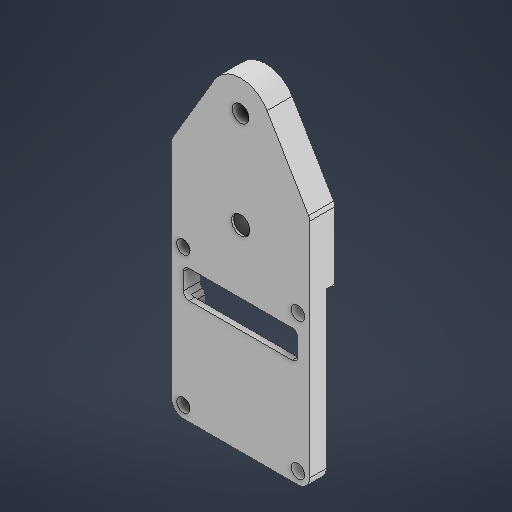
# Autodesk Inventor part: servo_side_plate2
Saved by Autodesk Inventor 2026 (Build 300175000, 175)
## iProperties
Created: 2025-12-05
Part Number: servo_side_plate2
Material: Generic
Document SubType Name: Modeling
Designer: numai
Density: 1 g/cm^3
Appearance: Default
Author: numai
Autodesk Inventor part; units mm, degrees
ref_plane "YZ Plane" through (0, 0, 0) normal (1, 0, 0) x (0, 1, 0)
ref_plane "XZ Plane" through (0, 0, 0) normal (0, 1, 0) x (-1, 0, 0)
ref_plane "XY Plane" through (0, 0, 0) normal (0, 0, 1) x (1, 0, 0)
sketch "スケッチ1" plane through (0, 0, 0) normal (0, 0, 1) x (1, 0, 0)
  circle A0 centre (0, 12.5) radius 5 construction
  line L0 (12.16, 19.2887) -> (12.16, 6.89) construction
  arc A1 (12.16, 19.2887) -> (11.7792, 20.2079) centre (10.86, 19.2887) ccw construction
  line L1 (9.9579, 22.0292) -> (11.7792, 20.2079) construction
  arc A2 (9.9579, 22.0292) -> (9.0387, 22.41) centre (9.0387, 21.11) ccw construction
  line L2 (0.95, 22.41) -> (9.0387, 22.41) construction
  line L3 (0.95, 19.61) -> (0.95, 22.41) construction
  arc A3 (-0.95, 19.61) -> (0.95, 19.61) centre (0, 19.61) ccw construction
  line L4 (-0.95, 22.41) -> (-0.95, 19.61) construction
  line L5 (-9.0387, 22.41) -> (-0.95, 22.41) construction
  arc A4 (-9.0387, 22.41) -> (-9.9579, 22.0292) centre (-9.0387, 21.11) ccw construction
  line L6 (-11.7792, 20.2079) -> (-9.9579, 22.0292) construction
  arc A5 (-11.7792, 20.2079) -> (-12.16, 19.2887) centre (-10.86, 19.2887) ccw construction
  line L7 (-12.16, 6.89) -> (-12.16, 19.2887) construction
  line L8 (-12.16, 6.89) -> (-9.9756, 6.89) construction
  arc A6 (-9.8028, 6.7907) -> (-9.9756, 6.89) centre (-9.9756, 6.69) ccw construction
  arc A7 (-9.8028, 6.7907) -> (-6.5643, 3.2479) centre (0, 12.5) ccw construction
  arc A8 (-6.48, 3.0847) -> (-6.5643, 3.2479) centre (-6.68, 3.0847) ccw construction
  line L9 (-6.48, 3.0847) -> (-6.48, 1.39) construction
  arc A9 (-6.68, 1.19) -> (-6.48, 1.39) centre (-6.68, 1.39) ccw construction
  line L10 (-6.68, 1.19) -> (6.68, 1.19) projected
  arc A10 (6.48, 1.39) -> (6.68, 1.19) centre (6.68, 1.39) ccw construction
  line L11 (6.48, 1.39) -> (6.48, 3.0847) construction
  arc A11 (6.5643, 3.2479) -> (6.48, 3.0847) centre (6.68, 3.0847) ccw construction
  arc A12 (6.5643, 3.2479) -> (9.8028, 6.7907) centre (0, 12.5) ccw construction
  arc A13 (9.9756, 6.89) -> (9.8028, 6.7907) centre (9.9756, 6.69) ccw construction
  line L12 (9.9756, 6.89) -> (12.16, 6.89) construction
  arc A14 (12.36, 19.2887) -> (12.1513, 20.052) centre (10.86, 19.2887) ccw projected
  arc A15 (-12.1513, 20.052) -> (-12.36, 19.2887) centre (-10.86, 19.2887) ccw projected
  line L13 (12.36, 19.2887) -> (12.36, -20.5) projected
  line L14 (-12.36, -20.5) -> (-12.36, 19.2887) projected
  line L15 (-12.36, 6.89) -> (-9.86, 6.89)
  line L16 (12.36, 6.89) -> (9.86, 6.89)
  arc A16 (-9.86, 6.89) -> (9.86, 6.89) centre (0, 12.5) ccw
  circle A17 centre (0, 12.5) radius 5.2
  arc A18 (4.7347, 32.5987) -> (-4.7347, 32.5987) centre (0, 29.8) ccw projected
  line L17 (-12.1513, 20.052) -> (-4.7347, 32.5987) projected
  circle A19 centre (0, 29.8) radius 1.5
  line L18 (4.7347, 32.5987) -> (12.1513, 20.052) projected
  circle A20 centre (0, 29.8) radius 1.5 construction
  point P0 (0, 0)
  point P1 (-11.1384, 22.2293)
  point P2 (11.1384, 22.2293)
  point P3 (-0.8807, 1.19)
  point P4 (0.8807, 1.19)
  dimension "d0" = 10.4
  constraints: 4 end point, 4 point on line, 3 centre point, 3 point on circle, 2 coincident, 2 concentric, 2 horizontal
  measures "d0" diameter of A17
extrude "押し出し1" add sketch "スケッチ1" along normal blind 1.5 contours A16 L15 L14 A15 L17 A18 L18 A14 L13 L16 L10
sketch "スケッチ2" plane through (0, 0, 1.5) normal (0, 0, 1) x (1, 0, 0)
  arc A0 (-9.86, 6.89) -> (-0.8807, 1.19) centre (0, 12.5) ccw projected
  line L0 (9.1914, -4.7213) -> (9.25, -4.7213) projected
  ellipse E0 centre (9.05, -4.9213) end of major axis (9.05, -4.6384) minor radius 0.2 (9.25, -4.9213) -> (9.1914, -4.7213) ccw projected
  line L1 (9.25, -4.9213) -> (9.25, -17.11) projected
  arc A1 (9.05, -17.31) -> (9.25, -17.11) centre (9.05, -17.11) ccw projected
  line L2 (9.05, -17.31) -> (-9.05, -17.31) projected
  arc A2 (-9.25, -17.11) -> (-9.05, -17.31) centre (-9.05, -17.11) ccw projected
  line L3 (-9.25, -17.11) -> (-9.25, -4.9213) projected
  ellipse E1 centre (-9.05, -4.9213) end of major axis (-9.05, -5.2041) minor radius 0.2 (-9.1914, -4.7213) -> (-9.25, -4.9213) ccw projected
  line L4 (-9.25, -4.7213) -> (-9.1914, -4.7213) projected
  ellipse E2 centre (-9.25, -3.0242) end of major axis (-9.25, -4.7213) minor radius 1.2 (-10.45, -3.0242) -> (-9.25, -4.7213) ccw projected
  line L5 (-10.45, 0.19) -> (-10.45, -3.0242) projected
  arc A3 (-9.25, 1.39) -> (-10.45, 0.19) centre (-9.25, 0.19) ccw projected
  line L6 (-6.68, 1.39) -> (-9.25, 1.39) projected
  line L7 (-6.68, 3.0847) -> (-6.68, 1.39) projected
  arc A4 (-9.9756, 6.69) -> (-6.68, 3.0847) centre (0, 12.5) ccw construction
  line L8 (-12.16, 6.69) -> (-9.9756, 6.69) construction
  line L9 (-12.16, -20.5) -> (-12.16, 6.69) construction
  arc A5 (-12.16, -20.5) -> (-10.25, -22.41) centre (-10.25, -20.5) ccw construction
  line L10 (10.25, -22.41) -> (-10.25, -22.41) construction
  arc A6 (10.25, -22.41) -> (12.16, -20.5) centre (10.25, -20.5) ccw construction
  line L11 (12.16, 6.69) -> (12.16, -20.5) construction
  line L12 (9.9756, 6.69) -> (12.16, 6.69) construction
  arc A7 (6.68, 3.0847) -> (9.9756, 6.69) centre (0, 12.5) ccw construction
  line L13 (6.68, 1.39) -> (6.68, 3.0847) projected
  line L14 (9.25, 1.39) -> (6.68, 1.39) projected
  arc A8 (10.45, 0.19) -> (9.25, 1.39) centre (9.25, 0.19) ccw projected
  line L15 (10.45, -3.0242) -> (10.45, 0.19) projected
  ellipse E3 centre (9.25, -3.0242) end of major axis (9.25, -4.7213) minor radius 1.2 (9.25, -4.7213) -> (10.45, -3.0242) ccw projected
  circle A9 centre (10.25, 4) radius 0.7835 construction
  circle A10 centre (10.25, -20.5) radius 0.7835 construction
  circle A11 centre (-10.25, -20.5) radius 0.7835 construction
  circle A12 centre (-10.25, 4) radius 0.7835 construction
  arc A13 (-12.36, -20.5) -> (-10.25, -22.61) centre (-10.25, -20.5) ccw projected
  line L16 (-12.36, 6.69) -> (-12.36, -20.5) projected
  line L17 (-10.25, -22.61) -> (10.25, -22.61) projected
  arc A14 (10.25, -22.61) -> (12.36, -20.5) centre (10.25, -20.5) ccw projected
  line L18 (12.36, -20.5) -> (12.36, 6.69) projected
  line L19 (12.36, 6.69) -> (12.36, 19.2887) projected
  line L20 (-12.36, 19.2887) -> (-12.36, 6.69) projected
  circle A15 centre (-10.25, 4) radius 1.2
  circle A16 centre (-10.25, -20.5) radius 1.2
  circle A17 centre (10.25, -20.5) radius 1.2
  circle A18 centre (10.25, 4) radius 1.2
  line L21 (-6.68, 3.0847) -> (-6.68, 3.3311)
  line L22 (6.68, 3.0847) -> (6.68, 3.3311)
  line L23 (-6.68, 1.39) -> (6.68, 1.39)
  line L24 (9.86, 6.89) -> (12.36, 6.89) projected
  line L25 (12.36, 6.89) -> (12.36, 19.2887) projected
  arc A19 (12.36, 19.2887) -> (12.1513, 20.052) centre (10.86, 19.2887) ccw projected
  line L26 (12.1513, 20.052) -> (4.7347, 32.5987) projected
  arc A20 (4.7347, 32.5987) -> (-4.7347, 32.5987) centre (0, 29.8) ccw projected
  line L27 (-4.7347, 32.5987) -> (-12.1513, 20.052) projected
  arc A21 (-12.1513, 20.052) -> (-12.36, 19.2887) centre (-10.86, 19.2887) ccw projected
  line L28 (-12.36, 19.2887) -> (-12.36, 6.89) projected
  line L29 (-12.36, 6.89) -> (-9.86, 6.89) projected
  line L30 (-0.8807, 1.19) -> (0.8807, 1.19) projected
  arc A22 (0.8807, 1.19) -> (9.86, 6.89) centre (0, 12.5) ccw projected
  circle A23 centre (0, 12.5) radius 5.2 projected
  circle A24 centre (0, 29.8) radius 1.5 projected
  arc A25 (-10.25, -2.81) -> (-9.25, -3.81) centre (-9.25, -2.81) ccw projected
  line L31 (-10.25, -3.0242) -> (-10.25, 0.19) projected
  arc A26 (-9.25, 1.19) -> (-10.25, 0.19) centre (-9.25, 0.19) ccw projected
  line L32 (-9.25, 1.19) -> (-6.68, 1.19) projected
  line L33 (-6.68, 1.19) -> (6.68, 1.19) projected
  line L34 (6.68, 1.19) -> (9.25, 1.19) projected
  arc A27 (10.25, 0.19) -> (9.25, 1.19) centre (9.25, 0.19) ccw projected
  line L35 (10.25, 0.19) -> (10.25, -3.0242) projected
  arc A28 (9.25, -3.81) -> (10.25, -2.81) centre (9.25, -2.81) ccw projected
  line L36 (-9.25, -3.81) -> (9.25, -3.81) projected
  line L37 (-9.25, -4.9213) -> (-9.25, -3.81)
  line L38 (9.25, -4.9213) -> (9.25, -3.81)
  point P0 (0, 0)
  point P1 (12.36, 6.89)
  point P2 (-2.2934, 1.39)
  point P3 (2.2934, 1.39)
  point P4 (2.2934, 1.39)
  dimension "d3" = 2.4
  constraints: 10 end point, 4 centre point, 4 coincident, 3 equal radius, 2 point on circle, 2 vertical, 1 horizontal, 1 parallel, 1 perpendicular, 1 point on line, 4 other
  measures "d3" diameter of A15
extrude "押し出し2" add sketch "スケッチ2" along normal blind 2 contours L29 L20 A21 L27 A20 L26 A19 L19 L24 A22 L23 A0 | A0 L21 L7 L6 A3 L5 E2 L37 L3 A2 L2 A1 L1 L38 E3 L15 A8 L14 L13 L22 A22 L24 L19 L18 A14 L17 A13 L16 L20 L29 | A0 L23 L7 L21 | L23 A22 L30 A0 | A0 L33 L32 A26 L31 A25 L37 E2 L5 A3 L6 L23 | A22 L22 L13 L23 | L23 L14 A8 L15 E3 L38 A28 L35 A27 L34 L33 A22
sketch "スケッチ3" plane through (0, 0, 3.5) normal (0, 0, 1) x (1, 0, 0)
  line L0 (-12.36, 19.2887) -> (-12.36, -20.5) projected
  arc A0 (-12.36, -20.5) -> (-10.25, -22.61) centre (-10.25, -20.5) ccw projected
  line L1 (-10.25, -22.61) -> (10.25, -22.61) projected
  arc A1 (10.25, -22.61) -> (12.36, -20.5) centre (10.25, -20.5) ccw projected
  line L2 (12.36, -20.5) -> (12.36, 19.2887) projected
  arc A2 (12.36, 19.2887) -> (12.1513, 20.052) centre (10.86, 19.2887) ccw projected
  line L3 (12.1513, 20.052) -> (4.7347, 32.5987) projected
  arc A3 (4.7347, 32.5987) -> (-4.7347, 32.5987) centre (0, 29.8) ccw projected
  line L4 (-4.7347, 32.5987) -> (-12.1513, 20.052) projected
  arc A4 (-12.1513, 20.052) -> (-12.36, 19.2887) centre (-10.86, 19.2887) ccw projected
  line L5 (-9.25, -17.11) -> (-9.25, -3.81) projected
  arc A5 (-9.25, -17.11) -> (-9.05, -17.31) centre (-9.05, -17.11) ccw projected
  line L6 (9.05, -17.31) -> (-9.05, -17.31) projected
  arc A6 (9.05, -17.31) -> (9.25, -17.11) centre (9.05, -17.11) ccw projected
  circle A7 centre (-10.25, -20.5) radius 1.2 projected
  circle A8 centre (-10.25, 4) radius 1.2 projected
  circle A9 centre (10.25, 4) radius 1.2 projected
  circle A10 centre (10.25, -20.5) radius 1.2 projected
  line L7 (9.25, -3.81) -> (9.25, -17.11) projected
  arc A11 (-10.25, -2.81) -> (-9.25, -3.81) centre (-9.25, -2.81) ccw projected
  line L8 (-10.25, -2.81) -> (-10.25, 0.19) projected
  arc A12 (-9.25, 1.19) -> (-10.25, 0.19) centre (-9.25, 0.19) ccw projected
  line L9 (-9.25, 1.19) -> (9.25, 1.19) projected
  arc A13 (10.25, 0.19) -> (9.25, 1.19) centre (9.25, 0.19) ccw projected
  line L10 (10.25, 0.19) -> (10.25, -2.81) projected
  arc A14 (9.25, -3.81) -> (10.25, -2.81) centre (9.25, -2.81) ccw projected
  circle A15 centre (0, 29.8) radius 1.5 projected
  circle A16 centre (0, 12.5) radius 5.2 projected
  line L11 (-9.25, -3.81) -> (9.25, -3.81)
  constraints: 2 end point, 1 horizontal, 1 tangent
extrude "押し出し3" add sketch "スケッチ3" along normal blind 1 contours A4 L4 A3 L3 A2 L2 A1 L1 A0 L0 | L5 L11 L7 A6 L6 A5
sketch "スケッチ5" plane through (0, 0, 4.5) normal (0, 0, 1) x (1, 0, 0)
  circle A0 centre (0, 12.5) radius 5.2382
  circle A1 centre (0, 12.5) radius 3.15
  point P0 (0, 0)
  dimension "d11" = 6.3
  constraints: 2 centre point, 1 coincident
  measures "d11" diameter of A1
extrude "押し出し5" add sketch "スケッチ5" against normal blind 4
sketch "スケッチ6" plane through (0, 0, 4.5) normal (0, 0, 1) x (1, 0, 0)
  circle A0 centre (0, 12.5) radius 3.15 projected
  circle A1 centre (0, 12.5) radius 1.65
  point P0 (0, 0)
  dimension "d14" = 3.3
  constraints: 1 centre point, 1 coincident
  measures "d14" diameter of A1
extrude "押し出し6" add sketch "スケッチ6" against normal blind 0.4
fillet "フィレット1" radius 0.4 2 edges at (-12.36, 6.89, 0.75) (12.36, 6.89, 0.75)
sketch "スケッチ7" plane through (0, 0, 0) normal (0, 0, -1) x (-1, 0, 0)
  circle A0 centre (0, 29.8) radius 1.5 projected
  circle A1 centre (0, 29.8) radius 3.9
  point P0 (0, 0)
  dimension "d18" = 7.8
  constraints: 1 centre point, 1 coincident
  measures "d18" diameter of A1
extrude "押し出し7" add sketch "スケッチ7" along normal blind 1
sketch "スケッチ8" plane through (0, 0, 3.5) normal (0, 0, -1) x (-1, 0, 0)
  line L0 (-9.25, -3.81) -> (-9.25, -17.11) projected
  arc A0 (-9.25, -17.11) -> (-9.05, -17.31) centre (-9.05, -17.11) ccw projected
  line L1 (-9.05, -17.31) -> (9.05, -17.31) projected
  arc A1 (9.05, -17.31) -> (9.25, -17.11) centre (9.05, -17.11) ccw projected
  line L2 (9.25, -17.11) -> (9.25, -3.81) projected
  line L3 (-9.25, -3.81) -> (9.25, -3.81) projected
  line L4 (9.35, -3.71) -> (9.35, -17.11)
  arc A2 (9.05, -17.41) -> (9.35, -17.11) centre (9.05, -17.11) ccw
  line L5 (9.05, -17.41) -> (-9.05, -17.41)
  arc A3 (-9.35, -17.11) -> (-9.05, -17.41) centre (-9.05, -17.11) ccw
  line L6 (-9.35, -17.11) -> (-9.35, -3.71)
  line L7 (-9.35, -3.71) -> (9.35, -3.71)
  point P0 (0, 0)
  dimension "d21" = 0.1
  constraints: 8 end point, 4 point on circle, 2 centre point, 5 other
  measures "d21" distance between parallel lines of L3 L7
extrude "押し出し8" cut sketch "スケッチ8" along normal through all
sketch "スケッチ10" plane through (0, 0, 1.5) normal (0, 0, -1) x (-1, 0, 0)
  line L0 (-9.35, -17.11) -> (-9.35, -3.805) projected
  arc A0 (-10.25, -2.81) -> (-9.35, -3.805) centre (-9.25, -2.81) ccw projected
  line L1 (-10.25, 0.19) -> (-10.25, -2.81) projected
  arc A1 (-9.25, 1.19) -> (-10.25, 0.19) centre (-9.25, 0.19) ccw projected
  arc A2 (-9.86, 6.89) -> (-0.8807, 1.19) centre (0, 12.5) ccw projected
  line L2 (-9.86, 6.89) -> (-11.96, 6.89) projected
  arc A3 (-12.36, 7.29) -> (-11.96, 6.89) centre (-11.96, 7.29) ccw projected
  line L3 (-12.36, -20.5) -> (-12.36, 7.29) projected
  arc A4 (-12.36, -20.5) -> (-10.25, -22.61) centre (-10.25, -20.5) ccw projected
  line L4 (10.25, -22.61) -> (-10.25, -22.61) projected
  arc A5 (10.25, -22.61) -> (12.36, -20.5) centre (10.25, -20.5) ccw projected
  line L5 (12.36, 7.29) -> (12.36, -20.5) projected
  arc A6 (11.96, 6.89) -> (12.36, 7.29) centre (11.96, 7.29) ccw projected
  line L6 (11.96, 6.89) -> (9.86, 6.89) projected
  arc A7 (0.8807, 1.19) -> (9.86, 6.89) centre (0, 12.5) ccw projected
  arc A8 (10.25, 0.19) -> (9.25, 1.19) centre (9.25, 0.19) ccw projected
  line L7 (10.25, -2.81) -> (10.25, 0.19) projected
  arc A9 (9.35, -3.805) -> (10.25, -2.81) centre (9.25, -2.81) ccw projected
  line L8 (9.35, -3.805) -> (9.35, -17.11) projected
  arc A10 (9.05, -17.41) -> (9.35, -17.11) centre (9.05, -17.11) ccw projected
  line L9 (9.05, -17.41) -> (-9.05, -17.41) projected
  arc A11 (-9.35, -17.11) -> (-9.05, -17.41) centre (-9.05, -17.11) ccw projected
  circle A12 centre (10.25, 4) radius 1.2 projected
  circle A13 centre (10.25, -20.5) radius 1.2 projected
  circle A14 centre (-10.25, -20.5) radius 1.2 projected
  circle A15 centre (-10.25, 4) radius 1.2 projected
  circle A16 centre (0, 12.5) radius 1.65 projected
  line L10 (0.8807, 1.19) -> (-0.8807, 1.19) projected
  arc A17 (-0.8807, 1.19) -> (0.8807, 1.19) centre (0, 12.5) ccw
  arc A18 (-9.8017, 6.99) -> (-0.8768, 1.29) centre (0, 12.5) ccw
  line L11 (-9.8017, 6.99) -> (-12.46, 6.99)
  line L12 (-12.46, 6.99) -> (-12.46, -20.5)
  arc A19 (-12.46, -20.5) -> (-10.25, -22.71) centre (-10.25, -20.5) ccw
  line L13 (-10.25, -22.71) -> (10.25, -22.71)
  arc A20 (10.25, -22.71) -> (12.46, -20.5) centre (10.25, -20.5) ccw
  line L14 (12.46, -20.5) -> (12.46, 6.99)
  line L15 (12.46, 6.99) -> (9.8017, 6.99)
  arc A21 (0.8768, 1.29) -> (9.8017, 6.99) centre (0, 12.5) ccw
  line L16 (0.8768, 1.29) -> (-0.8768, 1.29)
  point P0 (0, 0)
  point P1 (12.2246, 6.99)
  point P2 (-12.2246, 6.99)
  dimension "d24" = 0.1
  constraints: 21 centre point, 12 end point, 10 point on circle, 1 coincident, 9 other
  measures "d24" distance between parallel lines of L3 L12
extrude "押し出し9" cut sketch "スケッチ10" along normal through all
sketch "スケッチ11" plane through (0, 0, 0) normal (0, 0, -1) x (-1, 0, 0)
  line L0 (-0.8768, 1.29) -> (0.8768, 1.29) projected
  arc A0 (-9.8017, 6.99) -> (-0.8768, 1.29) centre (0, 12.5) ccw projected
  arc A1 (0.8768, 1.29) -> (9.8017, 6.99) centre (0, 12.5) ccw projected
  circle A2 centre (0, 12.5) radius 3.15 projected
  arc A3 (-0.8768, 1.29) -> (0.8768, 1.29) centre (0, 12.5) ccw
  point P0 (0, 0)
  constraints: 2 point on circle, 1 centre point, 1 coincident
extrude "押し出し10" add sketch "スケッチ11" against normal up to surface (1.5 mm away) contours L0 A3
sketch "スケッチ15" plane through (0, 0, 0) normal (0, 0, -1) x (-1, 0, 0)
  arc A0 (-9.8017, 6.99) -> (9.8017, 6.99) centre (0, 12.5) ccw projected
  arc A1 (-9.3401, 6.99) -> (9.3401, 6.99) centre (0, 12.5) ccw
  line L0 (-9.8017, 6.99) -> (-9.3401, 6.99)
  line L1 (9.8017, 6.99) -> (12.2246, 6.99) projected
  line L2 (9.3401, 6.99) -> (9.8017, 6.99)
  point P0 (0, 0)
  dimension "d42" = 0.4
  constraints: 4 end point, 2 horizontal, 2 point on circle, 1 centre point
  measures "d42" radial gap between concentric circles of A0 A1
extrude "押し出し13" cut sketch "スケッチ15" against normal up to surface (1.5 mm away)
fillet "フィレット2" radius 1 2 edges at (9.35, -3.805, 2.5) (-9.35, -3.805, 2.5)
sketch "スケッチ13" plane through (0, 0, 4.5) normal (0, 0, 1) x (1, 0, 0)
  circle A0 centre (0, 29.8) radius 1.5 projected
  circle A1 centre (0, 29.5) radius 3
  point P0 (0, 0)
  dimension "d36" = 6
  constraints: 1 centre point, 1 vertical alignment
  measures "d36" diameter of A1
